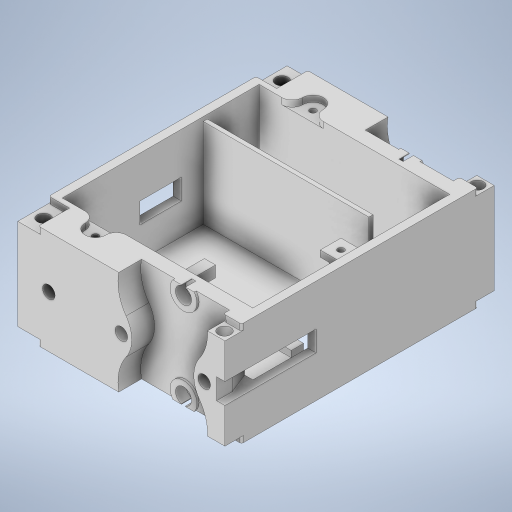
# Autodesk Inventor part: Body_2
Saved by Autodesk Inventor 2024 (Build 280153000, 153)
## iProperties
Created: 2024-04-13
Part Number: Body_2
Material: Generic
Document SubType Name: Modeling
Designer: CJ110
Density: 1 g/cm^3
Appearance: Default
Author: CJ110
Autodesk Inventor part; units mm, degrees
ref_plane "YZ Plane" through (0, 0, 0) normal (1, 0, 0) x (0, 1, 0)
ref_plane "XZ Plane" through (0, 0, 0) normal (0, 1, 0) x (-1, 0, 0)
ref_plane "XY Plane" through (0, 0, 0) normal (0, 0, 1) x (1, 0, 0)
sketch "Sketch1" plane through (0, 0, 0) normal (0, 0, 1) x (1, 0, 0)
  line L0 (0, 0) -> (-100, 0)
  line L1 (-100, 0) -> (-100, 50)
  line L2 (-100, 50) -> (0, 50)
  line L3 (0, 50) -> (0, 0)
  dimension "d0" = 50
  dimension "d1" = 100
  constraints: 8 end point, 2 parallel, 1 horizontal, 1 perpendicular
  measures "d0" distance of L2.end L0.start
  measures "d1" distance of L0.start L0.end
extrude "Extrusion1" add sketch "Sketch1" against normal blind 130
ref_plane "Work Plane1" through (-100, 25, 0) normal (0, 1, 0) x (1, 0, 0)
ref_plane "Work Plane2" through (0, 0, -65) normal (0, 0, -1) x (-1, 0, 0)
sketch "Sketch4" plane through (0, 0, 0) normal (0, 0, 1) x (1, 0, 0)
  circle A0 centre (-30, 46) radius 3.85
  circle A1 centre (-30, 4) radius 3.85
  line L0 (-120, 25) -> (20, 25) projected
  line L1 (0, 0) -> (0, 50) projected
  line L2 (-29, 50) -> (-29, 49.7179)
  line L3 (-31, 49.7179) -> (-31, 50)
  line L4 (0, 50) -> (-100, 50) projected
  line L5 (-100, 50) -> (-100, 0) projected
  line L6 (-100, 0) -> (0, 0) projected
  line L7 (0, 0) -> (0, 50) projected
  line L8 (-31, 0.2821) -> (-31, 0)
  line L9 (-29, 0.2821) -> (-29, 0)
  dimension "d6" = 42
  dimension "d7" = 7.7
  dimension "d8" = 21
  dimension "d11" = 30
  dimension "d17" = 1
  dimension "d18" = 2
  constraints: 8 end point, 4 point on circle, 4 point on line, 2 centre point, 2 collinear, 2 perpendicular, 1 equal radius, 1 parallel, 1 vertical, 1 vertical alignment
  measures "d6" distance of A1.centre A0.centre
  measures "d7" diameter of A0
  measures "d8" distance from line of L0 A0.centre
  measures "d11" distance from line of L1 A0.centre
  measures "d17" distance from line of A0.centre L3
  measures "d18" distance between parallel lines of L3 L2
extrude "Extrusion2" cut sketch "Sketch4" against normal blind 15 contours A0 | A0 L3 L4 L2 | L6 L8 A1 L9 | A1
sketch "Sketch3" plane through (0, 0, 0) normal (0, 0, 1) x (1, 0, 0)
  circle A0 centre (-60, 25) radius 15
  circle A1 centre (0, 25) radius 15
  line L0 (-123, 25) -> (38, 25) projected
  line L1 (0, 0) -> (0, 50) projected
  line L2 (0, 50) -> (-29, 50) projected
  line L3 (-100, 50) -> (-100, 0) projected
  line L4 (-100, 0) -> (-31, 0) projected
  line L5 (0, 0) -> (0, 50) projected
  arc A2 (-51.2464, 50) -> (-47.7115, 33.6019) centre (-30, 46) ccw
  arc A3 (-12.2885, 33.6019) -> (-8.7536, 50) centre (-30, 46) ccw
  arc A4 (-8.7536, 0) -> (-12.2885, 16.3981) centre (-30, 4) ccw
  arc A5 (-47.7115, 16.3981) -> (-51.2464, 0) centre (-30, 4) ccw
  line L6 (-29, 0.2821) -> (-29, 0) projected
  line L7 (-29, 0) -> (0, 0) projected
  line L8 (-29, 50) -> (-29, 49.7179) projected
  arc A6 (-31, 49.7179) -> (-29, 49.7179) centre (-30, 46) ccw projected
  line L9 (-31, 49.7179) -> (-31, 50) projected
  line L10 (-31, 50) -> (-100, 50) projected
  line L11 (-31, 0) -> (-31, 0.2821) projected
  arc A7 (-29, 0.2821) -> (-31, 0.2821) centre (-30, 4) ccw projected
  point P0 (-8.7536, 0)
  point P1 (0, 40)
  point P2 (0, 10)
  dimension "d4" = 30
  dimension "d5" = 60
  dimension "d14" = 42
  dimension "d20" = 21
  constraints: 12 point on circle, 6 centre point, 6 point on line, 4 tangent, 3 equal radius, 2 coincident, 1 midpoint
  measures "d4" diameter of A0
  measures "d5" distance of A0.centre A1.centre
  measures "d14" distance of A4.centre A2.centre
  measures "d20" distance from line of L0 A2.centre
extrude "Extrusion3" cut sketch "Sketch3" against normal blind 11 contours L0 A1 A4 L7 L6 A7 L11 L4 A5 A0 | A0 A2 L10 L9 A6 L8 L2 A3 A1 L0
sketch "Sketch5" plane through (0, 0, -11) normal (0, 0, 1) x (1, 0, 0)
  circle A0 centre (-30, 46) radius 6.5
  circle A1 centre (-30, 4) radius 6.5
  arc A2 (-31, 49.7179) -> (-29, 49.7179) centre (-30, 46) ccw projected
  line L0 (-31, 50) -> (-31, 49.7179) projected
  line L1 (-51.2464, 50) -> (-31, 50) projected
  arc A3 (-51.2464, 50) -> (-47.7115, 33.6019) centre (-30, 46) ccw projected
  arc A4 (-47.7115, 16.3981) -> (-47.7115, 33.6019) centre (-60, 25) ccw projected
  arc A5 (-47.7115, 16.3981) -> (-51.2464, 0) centre (-30, 4) ccw projected
  line L2 (-31, 0) -> (-51.2464, 0) projected
  line L3 (-31, 0.2821) -> (-31, 0) projected
  arc A6 (-29, 0.2821) -> (-31, 0.2821) centre (-30, 4) ccw projected
  line L4 (-29, 0) -> (-29, 0.2821) projected
  line L5 (-8.7536, 0) -> (-29, 0) projected
  arc A7 (-8.7536, 0) -> (-12.2885, 16.3981) centre (-30, 4) ccw projected
  arc A8 (-12.2885, 33.6019) -> (-12.2885, 16.3981) centre (0, 25) ccw projected
  arc A9 (-12.2885, 33.6019) -> (-8.7536, 50) centre (-30, 46) ccw projected
  line L6 (-29, 50) -> (-8.7536, 50) projected
  line L7 (-29, 49.7179) -> (-29, 50) projected
  line L8 (0, 0) -> (0, 50) projected
  line L9 (-120, 25) -> (20, 25) projected
  point P0 (-24.8765, 0)
  point P1 (-35.1235, 0)
  point P2 (-35.1235, 50)
  point P3 (-24.8765, 50)
  dimension "d19" = 42
  dimension "d21" = 30
  dimension "d22" = 13
  dimension "d23" = 21
  constraints: 2 centre point, 1 equal radius, 1 vertical alignment
  measures "d19" distance of A0.centre A1.centre
  measures "d21" distance from line of L8 A0.centre
  measures "d22" diameter of A0
  measures "d23" distance from line of L9 A0.centre
extrude "Extrusion4" add sketch "Sketch5" along normal blind 1 contours A0 L1 L0 A2 L7 L6 | L5 L4 A6 L3 L2 A1 picked at (-34.7492, 48.9391) picked at (-34.7492, 1.0609)
mirror "Mirror1" about plane through (0, 0, -65) normal (0, 0, -1) of "Extrusion4", "Extrusion3", "Extrusion2"
sketch "Sketch6" plane through (0, 0, 0) normal (0, 0, 1) x (1, 0, 0)
  arc A0 (-47.7115, 16.3981) -> (-51.2464, 0) centre (-30, 4) ccw projected
  arc A1 (-47.7115, 16.3981) -> (-47.7115, 33.6019) centre (-60, 25) ccw projected
  arc A2 (-51.2464, 50) -> (-47.7115, 33.6019) centre (-30, 46) ccw projected
  line L0 (-51.2464, 50) -> (-100, 50) projected
  line L1 (-100, 50) -> (-100, 0) projected
  line L2 (-100, 0) -> (-51.2464, 0) projected
  arc A3 (-8.7536, 0) -> (-12.2885, 16.3981) centre (-30, 4) ccw projected
  line L3 (-8.7536, 0) -> (0, 0) projected
  line L4 (0, 0) -> (0, 50) projected
  line L5 (0, 50) -> (-8.7536, 50) projected
  arc A4 (-12.2885, 33.6019) -> (-8.7536, 50) centre (-30, 46) ccw projected
  arc A5 (-12.2885, 33.6019) -> (-12.2885, 16.3981) centre (0, 25) ccw projected
  circle A6 centre (-50, 25) radius 3
  circle A7 centre (-10, 25) radius 3
  line L6 (-120, 25) -> (20, 25) projected
  circle A8 centre (-85, 25) radius 3
  dimension "d26" = 6
  dimension "d27" = 40
  dimension "d28" = 20
  dimension "d29" = 15
  constraints: 3 centre point, 2 equal radius, 2 point on line, 1 midpoint
  measures "d26" diameter of A8
  measures "d27" distance of A7.centre A6.centre
  measures "d28" horizontal distance of A2.centre A7.centre
  measures "d29" distance from line of L1 A8.centre
extrude "Extrusion5" cut sketch "Sketch6" against normal blind 10 contours L6 A6 | A6 L6 | A8 L6 | L6 A8 | L6 A7 | A7 L6
mirror "Mirror2" about plane through (0, 0, -65) normal (0, 0, -1) of "Extrusion5"
sketch "Sketch7" plane through (0, 0, 0) normal (0, 0, 1) x (1, 0, 0)
  circle A0 centre (-10, 25) radius 3 projected
  arc A1 (-8.7536, 0) -> (-12.2885, 16.3981) centre (-30, 4) ccw projected
  line L0 (-8.7536, 0) -> (0, 0) projected
  line L1 (0, 0) -> (0, 50) projected
  line L2 (0, 50) -> (-8.7536, 50) projected
  arc A2 (-12.2885, 33.6019) -> (-8.7536, 50) centre (-30, 46) ccw projected
  arc A3 (-12.2885, 33.6019) -> (-12.2885, 16.3981) centre (0, 25) ccw projected
  line L3 (-8.4035, 47) -> (0, 47)
  line L4 (-8.4035, 3) -> (0, 3)
  dimension "d32" = 3
  dimension "d33" = 3
  constraints: 4 end point, 2 perpendicular, 2 point on circle, 2 point on line
  measures "d32" distance between parallel lines of L2 L3
  measures "d33" distance between parallel lines of L0 L4
extrude "Extrusion6" cut sketch "Sketch7" against normal blind 8 contours A1 L4 L1 L0 | L3 A2 L2 L1
sketch "Sketch8" plane through (0, 0, 0) normal (0, 0, 1) x (1, 0, 0)
  circle A0 centre (-85, 25) radius 3 projected
  circle A1 centre (-50, 25) radius 3 projected
  arc A2 (-47.7115, 16.3981) -> (-51.2464, 0) centre (-30, 4) ccw projected
  arc A3 (-47.7115, 16.3981) -> (-47.7115, 33.6019) centre (-60, 25) ccw projected
  arc A4 (-51.2464, 50) -> (-47.7115, 33.6019) centre (-30, 46) ccw projected
  line L0 (-51.2464, 50) -> (-100, 50) projected
  line L1 (-100, 50) -> (-100, 0) projected
  line L2 (-100, 0) -> (-51.2464, 0) projected
  line L3 (-100, 47) -> (-90, 47)
  line L4 (-90, 47) -> (-90, 50)
  line L5 (-90, 50) -> (-100, 50)
  line L6 (-100, 50) -> (-100, 47)
  line L7 (-100, 0) -> (-90, 0)
  line L8 (-90, 0) -> (-90, 3)
  line L9 (-90, 3) -> (-100, 3)
  line L10 (-100, 3) -> (-100, 0)
  point P0 (0, 0)
  dimension "d36" = 10
  dimension "d37" = 10
  dimension "d38" = 3
  dimension "d39" = 3
  constraints: 16 end point, 4 parallel, 2 horizontal, 2 perpendicular, 2 point on line
  measures "d36" distance between parallel lines of L1 L8
  measures "d37" distance between parallel lines of L1 L4
  measures "d38" distance between parallel lines of L0 L3
  measures "d39" distance between parallel lines of L2 L9
extrude "Extrusion7" cut sketch "Sketch8" against normal blind 15 contours L2 L1 L9 L8 | L4 L3 L1 L0
sketch "Sketch9" plane through (-100, 47, 0) normal (0, 1, 0) x (1, 0, 0)
  line L0 (10, 0) -> (0, 0) projected
  line L1 (10, 0) -> (10, 15) projected
  line L2 (10, 15) -> (0, 15) projected
  line L3 (0, 0) -> (0, 15) projected
  line L4 (100, 0) -> (91.5965, 0) projected
  line L5 (100, 8) -> (100, 0) projected
  line L6 (100, 8) -> (91.5965, 8) projected
  line L7 (91.5965, 0) -> (91.5965, 8) projected
  circle A0 centre (5, 7.5) radius 3
  circle A1 centre (95.7983, 4) radius 3
  line L8 (95.7983, 0) -> (95.7983, 8) construction
  line L9 (91.5965, 4) -> (100, 4) construction
  line L10 (0, 7.5) -> (10, 7.5) construction
  line L11 (5, 15) -> (5, 0) construction
  point P0 (100, 0)
  dimension "d42" = 6
  dimension "d43" = 6
  constraints: 10 midpoint, 8 end point, 2 centre point
  measures "d42" diameter of A0
  measures "d43" diameter of A1
extrude "Extrusion8" cut sketch "Sketch9" against normal blind 11 contours A1
extrude "Extrusion9" cut sketch "Sketch9" against normal blind 5 contours A0
mirror "Mirror3" about plane through (-100, 25, 0) normal (0, 1, 0) of "Extrusion8", "Extrusion9"
mirror "Mirror4" about plane through (0, 0, -65) normal (0, 0, -1) of "Extrusion8", "Extrusion9", "Mirror3", "Extrusion7", "Extrusion6"
sketch "Sketch10" plane through (-51.2464, 50, 0) normal (0, 1, 0) x (1, 0, 0)
  line L0 (51.2464, 122) -> (42.4928, 122) projected
  line L1 (42.4928, 122) -> (42.4928, 119) projected
  line L2 (42.4928, 119) -> (26.3699, 119) projected
  line L3 (26.3699, 119) -> (26.3699, 120) projected
  line L4 (26.3699, 120) -> (22.2464, 120) projected
  line L5 (22.2464, 120) -> (22.2464, 115) projected
  line L6 (22.2464, 115) -> (20.2464, 115) projected
  line L7 (20.2464, 115) -> (20.2464, 120) projected
  line L8 (20.2464, 120) -> (16.1229, 120) projected
  line L9 (16.1229, 119) -> (16.1229, 120) projected
  line L10 (16.1229, 119) -> (0, 119) projected
  line L11 (0, 119) -> (0, 130) projected
  line L12 (-38.7536, 130) -> (0, 130) projected
  line L13 (-38.7536, 130) -> (-38.7536, 115) projected
  line L14 (-38.7536, 115) -> (-48.7536, 115) projected
  line L15 (-48.7536, 15) -> (-48.7536, 115) projected
  line L16 (-48.7536, 15) -> (-38.7536, 15) projected
  line L17 (-38.7536, 15) -> (-38.7536, 0) projected
  line L18 (0, 0) -> (-38.7536, 0) projected
  line L19 (0, 0) -> (0, 11) projected
  line L20 (0, 11) -> (16.1229, 11) projected
  line L21 (16.1229, 11) -> (16.1229, 10) projected
  line L22 (20.2464, 10) -> (16.1229, 10) projected
  line L23 (20.2464, 10) -> (20.2464, 15) projected
  line L24 (20.2464, 15) -> (22.2464, 15) projected
  line L25 (22.2464, 15) -> (22.2464, 10) projected
  line L26 (26.3699, 10) -> (22.2464, 10) projected
  line L27 (26.3699, 11) -> (26.3699, 10) projected
  line L28 (26.3699, 11) -> (42.4928, 11) projected
  line L29 (42.4928, 11) -> (42.4928, 8) projected
  line L30 (42.4928, 8) -> (51.2464, 8) projected
  line L31 (51.2464, 8) -> (51.2464, 122) projected
  line L32 (-44.7536, 112.5) -> (47.2464, 112.5)
  line L33 (47.2464, 112.5) -> (47.2464, 17.5)
  line L34 (47.2464, 17.5) -> (-44.7536, 17.5)
  line L35 (-44.7536, 17.5) -> (-44.7536, 112.5)
  line L36 (-68.7536, 65) -> (71.2464, 65) projected
  line L37 (-44.7536, 112.5) -> (-48.7536, 112.5) construction
  line L38 (47.2464, 112.5) -> (51.2464, 112.5) construction
  point P0 (51.2464, 0)
  dimension "d48" = 92
  dimension "d49" = 95
  dimension "d50" = 47.5
  constraints: 12 end point, 3 point on line, 2 parallel, 2 perpendicular, 1 collinear, 1 horizontal
  measures "d48" distance of L32.start L32.end
  measures "d49" distance of L32.end L33.end
  measures "d50" distance between parallel lines of L36 L32
extrude "Extrusion10" cut sketch "Sketch10" against normal blind 45 contours L36 L35 L32 L33 | L33 L34 L35 L36
sketch "Sketch11" plane through (0, 3, 0) normal (1, 0, 0) x (0, 0, -1)
  line L0 (130, 44) -> (122, 44) projected
  line L1 (122, 44) -> (122, 47) projected
  line L2 (8, 47) -> (122, 47) projected
  line L3 (8, 47) -> (8, 44) projected
  line L4 (8, 44) -> (0, 44) projected
  line L5 (0, 0) -> (0, 44) projected
  line L6 (0, 0) -> (8, 0) projected
  line L7 (8, 0) -> (8, -3) projected
  line L8 (8, -3) -> (122, -3) projected
  line L9 (122, -3) -> (122, 0) projected
  line L10 (122, 0) -> (130, 0) projected
  line L11 (130, 44) -> (130, 0) projected
  line L12 (0, 27) -> (44, 27)
  line L13 (44, 27) -> (44, 17)
  line L14 (44, 17) -> (0, 17)
  line L15 (0, 17) -> (0, 27)
  line L16 (-26, 22) -> (156, 22) projected
  point P0 (0, -3)
  point P1 (0, 17)
  dimension "d53" = 44
  dimension "d54" = 10
  dimension "d55" = 5
  constraints: 8 end point, 2 parallel, 1 horizontal, 1 perpendicular, 1 point on line
  measures "d53" distance between parallel lines of L13 L15
  measures "d54" distance between parallel lines of L12 L14
  measures "d55" distance between parallel lines of L16 L12
extrude "Extrusion11" cut sketch "Sketch11" against normal up to surface (4 mm away) contours L16 L5 L12 L13 | L13 L14 L5 L16
sketch "Sketch12" plane through (-51.2464, 50, 0) normal (0, 1, 0) x (1, 0, 0)
  line L0 (47.2464, 17.5) -> (-44.7536, 17.5) projected
  line L1 (-44.7536, 17.5) -> (-44.7536, 112.5) projected
  line L2 (-44.7536, 112.5) -> (47.2464, 112.5) projected
  line L3 (47.2464, 112.5) -> (47.2464, 17.5) projected
  line L4 (51.2464, 122) -> (42.4928, 122) projected
  line L5 (42.4928, 122) -> (42.4928, 119) projected
  line L6 (42.4928, 119) -> (26.3699, 119) projected
  line L7 (26.3699, 119) -> (26.3699, 120) projected
  line L8 (26.3699, 120) -> (22.2464, 120) projected
  line L9 (22.2464, 120) -> (22.2464, 115) projected
  line L10 (22.2464, 115) -> (20.2464, 115) projected
  line L11 (20.2464, 115) -> (20.2464, 120) projected
  line L12 (20.2464, 120) -> (16.1229, 120) projected
  line L13 (16.1229, 119) -> (16.1229, 120) projected
  line L14 (16.1229, 119) -> (0, 119) projected
  line L15 (0, 119) -> (0, 130) projected
  line L16 (-38.7536, 130) -> (0, 130) projected
  line L17 (-38.7536, 130) -> (-38.7536, 115) projected
  line L18 (-38.7536, 115) -> (-48.7536, 115) projected
  line L19 (-48.7536, 15) -> (-48.7536, 115) projected
  line L20 (-48.7536, 15) -> (-38.7536, 15) projected
  line L21 (-38.7536, 15) -> (-38.7536, 0) projected
  line L22 (0, 0) -> (-38.7536, 0) projected
  line L23 (0, 0) -> (0, 11) projected
  line L24 (0, 11) -> (16.1229, 11) projected
  line L25 (16.1229, 11) -> (16.1229, 10) projected
  line L26 (20.2464, 10) -> (16.1229, 10) projected
  line L27 (20.2464, 10) -> (20.2464, 15) projected
  line L28 (20.2464, 15) -> (22.2464, 15) projected
  line L29 (22.2464, 15) -> (22.2464, 10) projected
  line L30 (26.3699, 10) -> (22.2464, 10) projected
  line L31 (26.3699, 11) -> (26.3699, 10) projected
  line L32 (26.3699, 11) -> (42.4928, 11) projected
  line L33 (42.4928, 11) -> (42.4928, 8) projected
  line L34 (42.4928, 8) -> (51.2464, 8) projected
  line L35 (51.2464, 8) -> (51.2464, 122) projected
  circle A0 centre (-23.7536, 117.5) radius 1.5
  circle A1 centre (-23.7536, 12.5) radius 1.5
  line L36 (-68.7536, 65) -> (71.2464, 65) projected
  point P0 (51.2464, 0)
  dimension "d58" = 25
  dimension "d59" = 25
  dimension "d60" = 3
  dimension "d61" = 3
  dimension "d62" = 105
  dimension "d63" = 52.5
  constraints: 2 centre point
  measures "d58" distance from line of L19 A1.centre
  measures "d59" distance from line of L19 A0.centre
  measures "d60" diameter of A0
  measures "d61" diameter of A1
  measures "d62" distance of A1.centre A0.centre
  measures "d63" distance from line of L36 A0.centre
extrude "Extrusion12" cut sketch "Sketch12" against normal blind 8 contours A0 | A1
sketch "Sketch13" plane through (-51.2464, 50, 0) normal (0, 1, 0) x (1, 0, 0)
  circle A0 centre (-23.7536, 12.5) radius 1.5 projected
  circle A1 centre (-23.7536, 117.5) radius 1.5 projected
  line L0 (47.2464, 17.5) -> (-44.7536, 17.5) projected
  line L1 (-44.7536, 17.5) -> (-44.7536, 112.5) projected
  line L2 (-44.7536, 112.5) -> (47.2464, 112.5) projected
  line L3 (47.2464, 112.5) -> (47.2464, 17.5) projected
  line L4 (51.2464, 122) -> (42.4928, 122) projected
  line L5 (42.4928, 122) -> (42.4928, 119) projected
  line L6 (42.4928, 119) -> (26.3699, 119) projected
  line L7 (26.3699, 119) -> (26.3699, 120) projected
  line L8 (26.3699, 120) -> (22.2464, 120) projected
  line L9 (22.2464, 120) -> (22.2464, 115) projected
  line L10 (22.2464, 115) -> (20.2464, 115) projected
  line L11 (20.2464, 115) -> (20.2464, 120) projected
  line L12 (20.2464, 120) -> (16.1229, 120) projected
  line L13 (16.1229, 119) -> (16.1229, 120) projected
  line L14 (16.1229, 119) -> (0, 119) projected
  line L15 (0, 119) -> (0, 130) projected
  line L16 (-38.7536, 130) -> (0, 130) projected
  line L17 (-38.7536, 130) -> (-38.7536, 115) projected
  line L18 (-38.7536, 115) -> (-48.7536, 115) projected
  line L19 (-48.7536, 15) -> (-48.7536, 115) projected
  line L20 (-48.7536, 15) -> (-38.7536, 15) projected
  line L21 (-38.7536, 15) -> (-38.7536, 0) projected
  line L22 (0, 0) -> (-38.7536, 0) projected
  line L23 (0, 0) -> (0, 11) projected
  line L24 (0, 11) -> (16.1229, 11) projected
  line L25 (16.1229, 11) -> (16.1229, 10) projected
  line L26 (20.2464, 10) -> (16.1229, 10) projected
  line L27 (20.2464, 10) -> (20.2464, 15) projected
  line L28 (20.2464, 15) -> (22.2464, 15) projected
  line L29 (22.2464, 15) -> (22.2464, 10) projected
  line L30 (26.3699, 10) -> (22.2464, 10) projected
  line L31 (26.3699, 11) -> (26.3699, 10) projected
  line L32 (26.3699, 11) -> (42.4928, 11) projected
  line L33 (42.4928, 11) -> (42.4928, 8) projected
  line L34 (42.4928, 8) -> (51.2464, 8) projected
  line L35 (51.2464, 8) -> (51.2464, 122) projected
  circle A2 centre (-23.7536, 12.5) radius 5
  circle A3 centre (-23.7536, 117.5) radius 5
  arc A4 (-13.7536, 17.5) -> (-18.7536, 12.5) centre (-13.7536, 12.5) ccw
  arc A5 (-28.7536, 12.5) -> (-33.7536, 17.5) centre (-33.7536, 12.5) ccw
  arc A6 (-33.7536, 112.5) -> (-28.7536, 117.5) centre (-33.7536, 117.5) ccw
  arc A7 (-18.7536, 117.5) -> (-13.7536, 112.5) centre (-13.7536, 117.5) ccw
  line L36 (-44.7536, 112.5) -> (47.2464, 112.5) projected
  line L37 (47.2464, 17.5) -> (-44.7536, 17.5) projected
  point P0 (51.2464, 0)
  dimension "d66" = 10
  constraints: 12 point on circle, 8 tangent, 6 centre point, 4 equal radius, 4 point on line, 2 coincident, 1 horizontal alignment
  measures "d66" diameter of A3
extrude "Extrusion13" cut sketch "Sketch13" against normal blind 3 contours A4 A2 L0 | A2 A5 L0 | A2 | L2 A3 A7 | L2 A6 A3 | A3
sketch "Sketch15" plane through (-4, 5, -17.5) normal (0, 0, -1) x (-1, 0, 0)
  line L0 (32, 40) -> (37.4, 40)
  line L1 (37.4, 40) -> (37.4, 34.6)
  line L2 (37.4, 34.6) -> (32, 34.6)
  line L3 (32, 34.6) -> (32, 40)
  line L4 (86.6, 5.4) -> (92, 5.4)
  line L5 (92, 5.4) -> (92, 0)
  line L6 (92, 0) -> (86.6, 0)
  line L7 (86.6, 0) -> (86.6, 5.4)
  line L8 (32, 5.4) -> (37.4, 5.4)
  line L9 (37.4, 5.4) -> (37.4, 0)
  line L10 (37.4, 0) -> (32, 0)
  line L11 (32, 0) -> (32, 5.4)
  circle A0 centre (89.3, 2.7) radius 1.5
  circle A1 centre (34.7, 2.7) radius 1.5
  circle A2 centre (34.7, 37.3) radius 1.5
  line L12 (34.7, 40) -> (34.7, 34.6) construction
  line L13 (32, 37.3) -> (37.4, 37.3) construction
  line L14 (34.7, 5.4) -> (34.7, 0) construction
  line L15 (32, 2.7) -> (37.4, 2.7) construction
  line L16 (86.6, 2.7) -> (92, 2.7) construction
  line L17 (89.3, 5.4) -> (89.3, 0) construction
  line L18 (61, 42) -> (61, 45) construction
  line L19 (0, 45) -> (61, 45) construction
  line L20 (0, 45) -> (0, 25) construction
  line L21 (0, 25) -> (0, 15) construction
  line L22 (0, 15) -> (0, 0) construction
  line L23 (0, 0) -> (92, 0) construction
  line L24 (92, 45) -> (92, 0) construction
  line L25 (81, 45) -> (92, 45) construction
  line L26 (81, 42) -> (81, 45) construction
  line L27 (81, 42) -> (61, 42) construction
  line L28 (0, 0) -> (92, 0) construction
  point P0 (-4, -5)
  dimension "d83" = 5.4
  dimension "d84" = 5.4
  dimension "d85" = 5.4
  dimension "d86" = 5.4
  dimension "d87" = 5.4
  dimension "d88" = 5.4
  dimension "d89" = 3
  dimension "d90" = 3
  dimension "d91" = 3
  dimension "d92" = 34.6
  dimension "d93" = 54.6
  dimension "d94" = 54.6
  constraints: 36 end point, 15 midpoint, 6 parallel, 3 centre point, 3 collinear, 3 horizontal, 3 perpendicular
  measures "d83" distance of L0.end L1.end
  measures "d84" distance of L1.end L2.end
  measures "d85" distance of L8.start L8.end
  measures "d86" distance of L8.end L9.end
  measures "d87" distance of L6.end L4.start
  measures "d88" distance of L4.start L4.end
  measures "d89" diameter of A2
  measures "d90" diameter of A1
  measures "d91" diameter of A0
  measures "d92" distance of A2.centre A1.centre
  measures "d93" distance of A0.centre A1.centre
  measures "d94" horizontal distance of A0.centre A2.centre
extrude "Extrusion15" add sketch "Sketch15" along normal blind 14
sketch "Sketch16" plane through (-4, 50, -112.5) normal (-1, 0, 0) x (0, 0, 1)
  line L0 (47.5, -60) -> (47.5, 10) projected
  line L1 (42.5, -2) -> (52.5, -2)
  line L2 (52.5, -2) -> (52.5, -11)
  line L3 (52.5, -11) -> (42.5, -11)
  line L4 (42.5, -11) -> (42.5, -2)
  line L5 (0, 0) -> (95, 0) projected
  point P0 (112.5, -50)
  dimension "d97" = 10
  dimension "d98" = 5
  dimension "d99" = 9
  dimension "d100" = 2
  constraints: 8 end point, 2 parallel, 1 horizontal, 1 perpendicular
  measures "d97" distance of L1.start L1.end
  measures "d98" distance from line of L0 L1.end
  measures "d99" distance of L1.end L2.end
  measures "d100" distance between parallel lines of L5 L1
extrude "Extrusion16" add sketch "Sketch16" along normal blind 10
sketch "Sketch17" plane through (-4, 39, -60) normal (0, 0, 1) x (1, 0, 0)
  line L0 (0, 9) -> (0, 0) projected
  line L1 (0, 9) -> (-10, 9) projected
  line L2 (-10, 0) -> (-10, 9) projected
  line L3 (0, 0) -> (-10, 0) projected
  line L4 (-10, 6) -> (-6, 6)
  line L5 (-6, 6) -> (0, 0)
  point P0 (4, -39)
  dimension "d103" = 3
  dimension "d104" = 6
  constraints: 4 end point, 1 horizontal, 1 point on line
  measures "d103" distance between parallel lines of L1 L4
  measures "d104" distance from line of L0 L4.end
extrude "Extrusion17" cut sketch "Sketch17" against normal up to surface (10 mm away) contours L3 L2 L4 L5
sketch "Sketch18" plane through (-4, 48, -60) normal (0, 1, 0) x (1, 0, 0)
  circle A0 centre (-5, 5) radius 1.5
  line L0 (0, 10) -> (0, 0) projected
  line L1 (0, 10) -> (-10, 10) projected
  line L2 (-10, 0) -> (-10, 10) projected
  line L3 (0, 0) -> (-10, 0) projected
  line L4 (0, 5) -> (-10, 5) construction
  line L5 (-5, 10) -> (-5, 0) construction
  point P0 (4, -60)
  dimension "d107" = 3
  constraints: 5 midpoint, 4 end point, 1 centre point
  measures "d107" diameter of A0
extrude "Extrusion18" cut sketch "Sketch18" against normal blind 10 contours A0
sketch "Sketch19" plane through (-51.2464, 5, 0) normal (0, 1, 0) x (1, 0, 0)
  line L0 (-44.7536, 31.5) -> (-39.3536, 31.5) projected
  line L1 (-39.3536, 31.5) -> (-39.3536, 17.5) projected
  line L2 (9.8464, 17.5) -> (-39.3536, 17.5) projected
  line L3 (9.8464, 17.5) -> (9.8464, 31.5) projected
  line L4 (9.8464, 31.5) -> (15.2464, 31.5) projected
  line L5 (15.2464, 31.5) -> (15.2464, 17.5) projected
  line L6 (47.2464, 17.5) -> (15.2464, 17.5) projected
  line L7 (47.2464, 112.5) -> (47.2464, 17.5) projected
  line L8 (-44.7536, 112.5) -> (47.2464, 112.5) projected
  line L9 (-44.7536, 31.5) -> (-44.7536, 112.5) projected
  line L10 (47.2464, 87.5) -> (-44.7536, 87.5)
  line L11 (47.2464, 85.5) -> (-44.7536, 85.5)
  line L12 (47.2464, 70) -> (37.2464, 70) projected
  point P0 (51.2464, 0)
  dimension "d110" = 2
  dimension "d111" = 15.5
  constraints: 4 end point, 4 point on line, 2 perpendicular
  measures "d110" distance between parallel lines of L10 L11
  measures "d111" distance between parallel lines of L12 L11
extrude "Extrusion19" add sketch "Sketch19" along normal blind 43 contours L9 L10 L7 L11
sketch "Sketch20" plane through (-96, 5, -85.5) normal (0, 0, 1) x (1, 0, 0)
  line L0 (92, 0) -> (0, 0) projected
  line L1 (92, 43) -> (92, 0) projected
  line L2 (0, 43) -> (92, 43) projected
  line L3 (0, 0) -> (0, 43) projected
  line L4 (80, 43) -> (90, 43)
  line L5 (90, 43) -> (90, 28)
  line L6 (90, 28) -> (80, 28)
  line L7 (80, 28) -> (80, 43)
  point P0 (96, -5)
  dimension "d114" = 10
  dimension "d115" = 15
  dimension "d116" = 2
  constraints: 8 end point, 2 parallel, 1 horizontal, 1 perpendicular, 1 point on line
  measures "d114" distance between parallel lines of L7 L5
  measures "d115" distance of L6.end L4.start
  measures "d116" distance between parallel lines of L1 L5
extrude "Extrusion20" cut sketch "Sketch20" against normal up to surface (2 mm away) contours L5 L6 L7 L2
sketch "Sketch21" plane through (-51.2464, 5, 0) normal (0, 1, 0) x (1, 0, 0)
  line L0 (32.2464, 73) -> (20.2464, 73)
  line L1 (20.2464, 73) -> (20.2464, 57)
  line L2 (20.2464, 57) -> (32.2464, 57)
  line L3 (32.2464, 57) -> (32.2464, 73)
  line L4 (-68.7536, 65) -> (71.2464, 65) projected
  line L5 (47.2464, 112.5) -> (47.2464, 17.5) projected
  point P0 (51.2464, 0)
  dimension "d119" = 16
  dimension "d120" = 12
  dimension "d121" = 8
  dimension "d122" = 15
  constraints: 8 end point, 2 parallel, 1 horizontal, 1 perpendicular
  measures "d119" distance of L2.end L0.start
  measures "d120" distance of L1.end L2.end
  measures "d121" distance between parallel lines of L4 L2
  measures "d122" distance between parallel lines of L5 L3
extrude "Extrusion21" cut sketch "Sketch21" against normal through all
sketch "Sketch22" plane through (-51.2464, 5, 0) normal (0, 1, 0) x (1, 0, 0)
  line L0 (32.2464, 57) -> (20.2464, 57) projected
  line L1 (20.2464, 57) -> (20.2464, 73) projected
  line L2 (20.2464, 73) -> (32.2464, 73) projected
  line L3 (32.2464, 73) -> (32.2464, 57) projected
  line L4 (47.2464, 85.5) -> (-44.7536, 85.5) projected
  line L5 (-44.7536, 31.5) -> (-44.7536, 85.5) projected
  line L6 (-44.7536, 31.5) -> (-39.3536, 31.5) projected
  line L7 (-39.3536, 31.5) -> (-39.3536, 17.5) projected
  line L8 (9.8464, 17.5) -> (-39.3536, 17.5) projected
  line L9 (9.8464, 17.5) -> (9.8464, 31.5) projected
  line L10 (9.8464, 31.5) -> (15.2464, 31.5) projected
  line L11 (15.2464, 31.5) -> (15.2464, 17.5) projected
  line L12 (47.2464, 17.5) -> (15.2464, 17.5) projected
  line L13 (47.2464, 85.5) -> (47.2464, 17.5) projected
  line L14 (32.2464, 57) -> (20.2464, 57)
  line L15 (20.2464, 57) -> (20.2464, 51)
  line L16 (20.2464, 51) -> (32.2464, 51)
  line L17 (32.2464, 51) -> (32.2464, 57)
  line L18 (32.2464, 73) -> (20.2464, 73)
  line L19 (20.2464, 73) -> (20.2464, 79)
  line L20 (20.2464, 79) -> (32.2464, 79)
  line L21 (32.2464, 79) -> (32.2464, 73)
  circle A0 centre (26.2464, 54.5) radius 1.5
  circle A1 centre (26.2464, 75.5) radius 1.5
  line L22 (26.2464, 79) -> (26.2464, 51) construction
  point P0 (51.2464, 0)
  point P1 (26.2464, 57)
  dimension "d125" = 6
  dimension "d126" = 3
  dimension "d127" = 3
  dimension "d128" = 2.5
  dimension "d129" = 2.5
  constraints: 18 end point, 4 parallel, 4 point on line, 3 midpoint, 2 centre point, 2 collinear, 2 horizontal, 2 perpendicular, 1 vertical
  measures "d125" distance of L16.end L0.start
  measures "d126" diameter of A0
  measures "d127" diameter of A1
  measures "d128" distance from line of L14 A0.centre
  measures "d129" distance from line of L2 A1.centre
extrude "Extrusion22" add sketch "Sketch22" along normal blind 3 contours L17 L16 L15 L0 | L2 L19 L20 L21
sketch "Sketch23" plane through (-100, 3, 0) normal (-1, 0, 0) x (0, 0, 1)
  line L0 (-115, 44) -> (-130, 44) projected
  line L1 (-130, 0) -> (-130, 44) projected
  line L2 (-130, 0) -> (-115, 0) projected
  line L3 (-115, 0) -> (-115, -3) projected
  line L4 (-15, -3) -> (-115, -3) projected
  line L5 (-15, -3) -> (-15, 0) projected
  line L6 (-15, 0) -> (0, 0) projected
  line L7 (0, 44) -> (0, 0) projected
  line L8 (0, 44) -> (-15, 44) projected
  line L9 (-15, 44) -> (-15, 47) projected
  line L10 (-15, 47) -> (-115, 47) projected
  line L11 (-115, 47) -> (-115, 44) projected
  line L12 (-75, 27) -> (-55, 27)
  line L13 (-55, 27) -> (-55, 17)
  line L14 (-55, 17) -> (-75, 17)
  line L15 (-75, 17) -> (-75, 27)
  line L16 (-156, 22) -> (26, 22) projected
  line L17 (-65, -13) -> (-65, 57) projected
  point P0 (0, -3)
  point P1 (-75, 22)
  point P2 (-65, 27)
  dimension "d132" = 20
  dimension "d133" = 10
  constraints: 8 end point, 2 midpoint, 2 parallel, 2 point on line, 1 horizontal, 1 perpendicular
  measures "d132" distance of L12.start L12.end
  measures "d133" distance of L12.end L13.end
extrude "Extrusion23" cut sketch "Sketch23" against normal up to surface (4 mm away) contours L16 L17 L14 L15 | L15 L12 L17 L16 | L12 L13 L16 L17 | L16 L13 L14 L17
chamfer "Chamfer1" distance 4 distance2 10 1 edges at (-4, 25, -17.5) measured on face at (-4.5, 25, -17.5)
fillet "Fillet1" radius 1 16 edges at (0, 48.5, -8) (-8.5261, 48.5061, -8) (-90, 48.5, 0) (-100, 48.5, -15) (0, 1.5, -8) (-8.5261, 1.4939, -8) (-100, 1.5, -15) (-90, 1.5, 0) (-90, 48.5, -130) (-100, 48.5, -115) (-100, 1.5, -115) (-90, 1.5, -130) (-8.5261, 48.5061, -122) (0, 48.5, -122) (0, 1.5, -122) (-8.5261, 1.4939, -122)
equation "\"d0\" = Body_Height"
equation "\"d1\" = Body_Length"
equation "\"d2\" = Body_Width"
equation "\"d6\" = SW_Dist_Apart"
equation "\"d7\" = SW_Hole_Diam"
equation "\"d8\" = 0.5 * d6"
equation "\"d17\" = 0.5 * d18"
equation "\"d12\" = SW_Hole_Depth"
equation "\"d5\" = 2 * SW_Dist_Front"
equation "\"d14\" = SW_Dist_Apart"
equation "\"d20\" = 0.5 * d14"
equation "\"d15\" = SW_Cavity_Depth"
equation "\"d19\" = SW_Dist_Apart"
equation "\"d21\" = SW_Dist_Front"
equation "\"d23\" = 0.5 * d19"
equation "\"d26\" = M4_Insert_Diam"
equation "\"d27\" = Arm_Screw_Distance"
equation "\"d28\" = 0.5 * d27"
equation "\"d29\" = DC_Hole_Dist_Back"
equation "\"d30\" = Arm_Hole_Depth"
equation "\"d32\" = Arm_Mount_Height"
equation "\"d33\" = Arm_Mount_Height"
equation "\"d34\" = Arm_Mount_Width"
equation "\"d36\" = DC_Mount_Depth"
equation "\"d37\" = DC_Mount_Depth"
equation "\"d38\" = Arm_Mount_Height"
equation "\"d39\" = Arm_Mount_Height"
equation "\"d40\" = DC_Mount_Width"
equation "\"d42\" = M4_Insert_Diam"
equation "\"d43\" = M4_Insert_Diam"
equation "\"d44\" = Arm_Mount_Hole_Depth"
equation "\"d46\" = DC_Mount_Hole_Depth"
equation "\"d48\" = Body_Cavity_Length"
equation "\"d49\" = Body_Cavity_Width"
equation "\"d50\" = 0.5 * d49"
equation "\"d51\" = Body_Cavity_Height"
equation "\"d53\" = BLDC_Wire_Cutout_Width"
equation "\"d54\" = BLDC_Wire_Cutout_Height"
equation "\"d55\" = 0.5 * d54"
equation "\"d56\" = Body_Cavity_Height"
equation "\"d58\" = Cover_Hole_Dist_Back"
equation "\"d59\" = Cover_Hole_Dist_Back"
equation "\"d60\" = M3_Screw_Diam"
equation "\"d61\" = M3_Screw_Diam"
equation "\"d62\" = Cover_Hole_Dist_Apart"
equation "\"d63\" = 0.5 * d62"
equation "\"d83\" = Board_Mount_Size"
equation "\"d84\" = Board_Mount_Size"
equation "\"d85\" = Board_Mount_Size"
equation "\"d86\" = Board_Mount_Size"
equation "\"d87\" = Board_Mount_Size"
equation "\"d88\" = Board_Mount_Size"
equation "\"d89\" = M3_Screw_Diam"
equation "\"d90\" = M3_Screw_Diam"
equation "\"d91\" = M3_Screw_Diam"
equation "\"d92\" = Board_Hole_Dist_Short"
equation "\"d93\" = Board_Hole_Dist_Long"
equation "\"d94\" = Board_Hole_Dist_Long"
equation "\"d95\" = Board_Mount_Depth"
equation "\"d98\" = 0.5 * d97"
equation "\"d107\" = M3_Screw_Diam"
equation "\"d110\" = Battery_Wall_Thickness"
equation "\"d112\" = Battery_Wall_Height"
equation "\"d117\" = Battery_Wall_Height"
equation "\"d119\" = Plug_Cuttout_Length"
equation "\"d120\" = Plug_Cuttout_Width"
equation "\"d121\" = 0.5 * d119"
equation "\"d126\" = M3_Screw_Diam"
equation "\"d127\" = M3_Screw_Diam"
equation "\"d129\" = d128"
equation "\"Body_Height\" = 50"
equation "\"Body_Length\" = 100"
equation "\"Body_Width\" = 130"
equation "\"SW_Hole_Diam\" = 7.7"
equation "\"SW_Dist_Front\" = 30"
equation "\"SW_Cavity_Depth\" = 11"
equation "\"SW_Hole_Depth\" = 15"
equation "\"M4_Insert_Diam\" = 6"
equation "\"M3_Screw_Diam\" = 3"
equation "\"Arm_Screw_Distance\" = 40"
equation "\"DC_Hole_Dist_Back\" = 15"
equation "\"Arm_Hole_Depth\" = 10"
equation "\"Arm_Mount_Height\" = 3"
equation "\"Arm_Mount_Width\" = 8"
equation "\"DC_Mount_Depth\" = 10"
equation "\"DC_Mount_Width\" = 15"
equation "\"Arm_Mount_Hole_Depth\" = 11"
equation "\"DC_Mount_Hole_Depth\" = 5"
equation "\"Body_Cavity_Length\" = 92"
equation "\"Body_Cavity_Width\" = 95"
equation "\"Body_Cavity_Height\" = 45"
equation "\"BLDC_Wire_Cutout_Width\" = 44"
equation "\"BLDC_Wire_Cutout_Height\" = 10"
equation "\"Cover_Hole_Dist_Back\" = 25"
equation "\"Cover_Hole_Dist_Apart\" = 105"
equation "\"Board_Mount_Size\" = 5.4"
equation "\"Board_Hole_Dist_Short\" = 34.6"
equation "\"Board_Hole_Dist_Long\" = 54.6"
equation "\"Board_Mount_Depth\" = 14"
equation "\"Battery_Wall_Thickness\" = 2"
equation "\"Battery_Wall_Height\" = 43"
equation "\"Plug_Cuttout_Length\" = 16"
equation "\"Plug_Cuttout_Width\" = 12"
equation "\"SW_Dist_Apart\" = 42"
body "Solid1"
